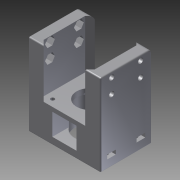
# Autodesk Inventor part: V5 Z Top
Saved by Autodesk Inventor 2012 (Build 160160000, 160)
## iProperties
Created: 2013-01-29
Part Number: V5 Z Top
Material: Default
Document SubType Name: Modeling
Designer: mce
Density: 1 g/cm^3
Author: mce
Autodesk Inventor part; units mm, degrees
ref_plane "YZ Plane" through (0, 0, 0) normal (1, 0, 0) x (0, 1, 0)
ref_plane "XZ Plane" through (0, 0, 0) normal (0, 1, 0) x (-1, 0, 0)
ref_plane "XY Plane" through (0, 0, 0) normal (0, 0, 1) x (1, 0, 0)
sketch "Sketch1" plane through (0, 0, 0) normal (0, 0, 1) x (1, 0, 0)
  line L0 (0, 0) -> (60, 0)
  line L1 (60, 0) -> (60, 42.4)
  line L2 (60, 42.4) -> (0, 42.4)
  line L3 (0, 42.4) -> (0, 0)
  line L4 (30, 50.4124) -> (30, -35.7574) construction
  line L5 (-22.9402, 21.2) -> (92.246, 21.2) construction
  circle A0 centre (30, 21.2) radius 11.1
  circle A1 centre (14.5, 36.7) radius 1.55
  circle A2 centre (45.5, 36.7) radius 1.55
  circle A3 centre (45.5, 5.7) radius 1.55
  circle A4 centre (14.5, 5.7) radius 1.55
  dimension "d0" = 60
  dimension "d1" = 42.4
  dimension "d2" = 22.2
  dimension "d3" = 3.1
  dimension "d4" = 31
  dimension "d5" = 31
  constraints: 12 end point, 5 centre point, 4 symmetric about line, 3 equal radius, 3 horizontal, 3 vertical, 2 point on line, 2 other
  measures "d0" distance of L0.start L0.end
  measures "d1" distance of L2.end L0.start
  measures "d2" diameter of A0
  measures "d3" diameter of A1
  measures "d4" distance of A4.centre A1.centre
  measures "d5" distance of A1.centre A2.centre
extrude "Extrusion1" add sketch "Sketch1" along normal blind 68
sketch "Sketch2" plane through (0, 0, 68) normal (0, 0, 1) x (1, 0, 0)
  circle A0 centre (30, 21.2) radius 11.1 projected
  circle A1 centre (14.5, 5.7) radius 1.55 projected
  circle A2 centre (45.5, 5.7) radius 1.55 projected
  circle A3 centre (45.5, 36.7) radius 1.55 projected
  circle A4 centre (14.5, 36.7) radius 1.55 projected
  line L0 (60, 0) -> (0, 0) projected
  line L1 (0, 42.4) -> (60, 42.4) projected
  line L2 (12.8, 42.4) -> (47.2, 42.4)
  line L3 (51.2, 38.4) -> (51.2, 4)
  line L4 (47.2, 0) -> (12.8, 0)
  line L5 (8.8, 4) -> (8.8, 38.4)
  line L6 (8.8, 38.4) -> (12.8, 42.4)
  line L7 (47.2, 42.4) -> (51.2, 38.4)
  line L8 (12.8, 0) -> (8.8, 4)
  line L9 (51.2, 4) -> (47.2, 0)
  point P0 (8.8, 42.4)
  point P1 (51.2, 0)
  point P2 (51.2, 42.4)
  point P3 (8.8, 0)
  dimension "d8" = 42.4
  dimension "d9" = 21.2
  dimension "d10" = 4
  dimension "d11" = 4
  dimension "d12" = 4
  dimension "d13" = 4
  dimension "d14" = 4
  dimension "d15" = 4
  dimension "d16" = 4
  dimension "d17" = 4
  constraints: 16 end point, 10 point on line
  measures "d8" distance between parallel lines of L5 L3
  measures "d9" distance from line of L5 A0.centre
  measures "d10" distance of L5.end point (8.8, 42.4)
  measures "d11" distance of L2.start point (8.8, 42.4)
  measures "d12" distance of L2.end point (51.2, 42.4)
  measures "d13" distance of L3.start point (51.2, 42.4)
  measures "d14" distance of L4.end point (8.8, 0)
  measures "d15" distance of L5.start point (8.8, 0)
  measures "d16" distance of L3.end point (51.2, 0)
  measures "d17" distance of L4.start point (51.2, 0)
extrude "Extrusion2" cut sketch "Sketch2" against normal blind 40.5
sketch "Sketch3" plane through (0, 0, 0) normal (-1, 0, 0) x (0, 0, 1)
  line L0 (68, 0) -> (68, 42.4) projected
  line L1 (0, 42.4) -> (68, 42.4) projected
  line L2 (0, 0) -> (68, 0) projected
  circle A0 centre (52, 33.2) radius 2.1
  circle A1 centre (64, 33.2) radius 2.1
  circle A2 centre (52, 9.2) radius 2.1
  circle A3 centre (64, 9.2) radius 2.1
  dimension "d20" = 4.2
  dimension "d21" = 12
  dimension "d22" = 12
  dimension "d23" = 4
  dimension "d24" = 9.2
  dimension "d25" = 9.2
  dimension "d26" = 4
  dimension "d27" = 9.2
  dimension "d28" = 9.2
  constraints: 4 centre point, 3 equal radius
  measures "d20" diameter of A0
  measures "d21" distance of A1.centre A0.centre
  measures "d22" distance of A2.centre A3.centre
  measures "d23" distance from line of L0 A1.centre
  measures "d24" distance from line of L1 A1.centre
  measures "d25" distance from line of L1 A0.centre
  measures "d26" distance from line of L0 A3.centre
  measures "d27" distance from line of L2 A3.centre
  measures "d28" distance from line of L2 A2.centre
extrude "Extrusion3" cut sketch "Sketch3" against normal through all
sketch "Sketch4" plane through (8.8, 4, 68) normal (1, 0, 0) x (0, 0, -1)
  circle A0 centre (4, 5.2) radius 2.1 projected
  circle A1 centre (16, 5.2) radius 2.1 projected
  circle A2 centre (4, 29.2) radius 2.1 projected
  circle A3 centre (16, 29.2) radius 2.1 projected
  line L0 (16, 25.1008) -> (12.45, 27.1504)
  line L1 (12.45, 27.1504) -> (12.45, 31.2496)
  line L2 (12.45, 31.2496) -> (16, 33.2992)
  line L3 (16, 33.2992) -> (19.55, 31.2496)
  line L4 (19.55, 31.2496) -> (19.55, 27.1504)
  line L5 (19.55, 27.1504) -> (16, 25.1008)
  line L6 (4, 25.1008) -> (0.45, 27.1504)
  line L7 (0.45, 27.1504) -> (0.45, 31.2496)
  line L8 (0.45, 31.2496) -> (4, 33.2992)
  line L9 (4, 33.2992) -> (7.55, 31.2496)
  line L10 (7.55, 31.2496) -> (7.55, 27.1504)
  line L11 (7.55, 27.1504) -> (4, 25.1008)
  line L12 (7.55, 3.1504) -> (4, 1.1008)
  line L13 (4, 1.1008) -> (0.45, 3.1504)
  line L14 (0.45, 3.1504) -> (0.45, 7.2496)
  line L15 (0.45, 7.2496) -> (4, 9.2992)
  line L16 (4, 9.2992) -> (7.55, 7.2496)
  line L17 (7.55, 7.2496) -> (7.55, 3.1504)
  line L18 (19.55, 3.1504) -> (16, 1.1008)
  line L19 (16, 1.1008) -> (12.45, 3.1504)
  line L20 (12.45, 3.1504) -> (12.45, 7.2496)
  line L21 (12.45, 7.2496) -> (16, 9.2992)
  line L22 (16, 9.2992) -> (19.55, 7.2496)
  line L23 (19.55, 7.2496) -> (19.55, 3.1504)
  point P0 (68, -4)
  point P1 (2.225, 26.1256)
  point P2 (12.45, 29.2)
  dimension "d31" = 7.1
  constraints: 48 end point, 4 coincident, 4 vertical, 3 equal length, 2 midpoint, 52 other
  measures "d31" distance between parallel lines of L16 L13
extrude "Extrusion4" cut sketch "Sketch4" against normal blind 5 and the other way blind 47.4
sketch "Sketch5" plane through (0, 1, 0) normal (-1, 0, 0) x (0, 0, 1)
  line L0 (0, 41.4) -> (0, -1) projected
  line L1 (7, 36) -> (10.5, 36)
  line L2 (10.5, 36) -> (10.5, 28.8)
  line L3 (10.5, 28.8) -> (7, 28.8)
  line L4 (7, 28.8) -> (7, 36)
  line L5 (7, 11.6) -> (10.5, 11.6)
  line L6 (10.5, 11.6) -> (10.5, 4.4)
  line L7 (10.5, 4.4) -> (7, 4.4)
  line L8 (7, 4.4) -> (7, 11.6)
  line L9 (0, 41.4) -> (68, 41.4) projected
  line L10 (68, 41.4) -> (27.5, 41.4) projected
  dimension "d37" = 7.2
  dimension "d38" = 3.5
  dimension "d39" = 24.4
  dimension "d41" = 7
  dimension "d105" = 5.4
  constraints: 16 end point, 4 vertical, 2 equal length, 2 horizontal, 1 collinear
  measures "d37" distance of L3.end L1.start
  measures "d38" distance of L1.start L1.end
  measures "d39" distance between parallel lines of L7 L3
  measures "d41" distance between parallel lines of L4 L0
  measures "d105" distance between parallel lines of L10 L1
extrude "Extrusion5" cut sketch "Sketch5" against normal blind 12
sketch "Sketch6" plane through (60, 1, 0) normal (1, 0, 0) x (0, 0, -1)
  line L0 (0, -1) -> (0, 41.4) projected
  line L1 (-10.5, 36) -> (-7, 36)
  line L2 (-7, 36) -> (-7, 28.8)
  line L3 (-7, 28.8) -> (-10.5, 28.8)
  line L4 (-10.5, 28.8) -> (-10.5, 36)
  line L5 (-10.5, 11.6) -> (-7, 11.6)
  line L6 (-7, 11.6) -> (-7, 4.4)
  line L7 (-7, 4.4) -> (-10.5, 4.4)
  line L8 (-10.5, 4.4) -> (-10.5, 11.6)
  line L9 (0, 41.4) -> (-68, 41.4) projected
  dimension "d44" = 3.5
  dimension "d45" = 7.2
  dimension "d46" = 7
  dimension "d47" = 24.4
  dimension "d67" = 5.4
  constraints: 16 end point, 4 horizontal, 4 vertical, 2 equal length, 1 collinear
  measures "d44" distance of L1.start L1.end
  measures "d45" distance of L1.end L2.end
  measures "d46" distance between parallel lines of L0 L2
  measures "d47" distance between parallel lines of L3 L7
  measures "d67" distance between parallel lines of L9 L1
extrude "Extrusion6" cut sketch "Sketch6" against normal blind 12
sketch "Sketch7" plane through (0, 0, 0) normal (0, 0, -1) x (-1, 0, 0)
  line L0 (-60, 0) -> (-60, 42.4) projected
  line L1 (0, 0) -> (-60, 0) projected
  line L2 (0, 42.4) -> (0, 0) projected
  line L3 (-60, 42.4) -> (0, 42.4) projected
  circle A0 centre (-55, 33.4) radius 2.05
  circle A1 centre (-5, 33.4) radius 2.05
  circle A2 centre (-5, 9) radius 2.05
  circle A3 centre (-55, 9) radius 2.05
  point P0 (-59, 42.4)
  point P1 (-60, 41.4)
  point P2 (-60, 1)
  point P3 (-59, 0)
  point P4 (-1, 0)
  point P5 (0, 1)
  point P6 (0, 41.4)
  point P7 (-1, 42.4)
  dimension "d51" = 5
  dimension "d52" = 5
  dimension "d53" = 5
  dimension "d54" = 5
  dimension "d55" = 9
  dimension "d56" = 9
  dimension "d57" = 9
  dimension "d58" = 9
  dimension "d59" = 4.1
  constraints: 4 centre point, 3 equal radius
  measures "d51" distance from line of L0 A0.centre
  measures "d52" distance from line of L0 A3.centre
  measures "d53" distance from line of L2 A2.centre
  measures "d54" distance from line of L2 A1.centre
  measures "d55" distance from line of L3 A0.centre
  measures "d56" distance from line of L1 A3.centre
  measures "d57" distance from line of L1 A2.centre
  measures "d58" distance from line of L3 A1.centre
  measures "d59" diameter of A0
extrude "Extrusion7" cut sketch "Sketch7" against normal blind 15 contours A0 | A1 | A2 | A3
sketch "Sketch8" plane through (0, 0, 0) normal (0, 0, -1) x (-1, 0, 0)
  circle A0 centre (-14.5, 5.7) radius 1.55 projected
  circle A1 centre (-45.5, 5.7) radius 1.55 projected
  circle A2 centre (-45.5, 36.7) radius 1.55 projected
  circle A3 centre (-14.5, 36.7) radius 1.55 projected
  circle A4 centre (-45.5, 36.7) radius 3
  circle A5 centre (-14.5, 36.7) radius 3
  circle A6 centre (-14.5, 5.7) radius 3
  circle A7 centre (-45.5, 5.7) radius 3
  point P0 (0, 0)
  dimension "d62" = 6
  constraints: 4 centre point, 4 coincident, 3 equal radius
  measures "d62" diameter of A4
extrude "Extrusion8" cut sketch "Sketch8" against normal blind 18
chamfer "Chamfer1" distance 3 angle 45 4 edges at (12, 12.6, 8.75) (12, 29.8, 8.75) (48, 29.8, 8.75) (48, 12.6, 8.75)
fillet "Fillet5" radius 3 2 edges at (53.6, 42.4, 68) (6.4, 42.4, 68)
fillet "Fillet3" radius 1 4 edges at (30, 42.4, 0) (60, 21.2, 0) (30, 0, 0) (0, 21.2, 0)
fillet "Fillet4" radius 1 10 edges at (60, 42.4, 33) (59.7071, 42.1071, 0.2929) (0.2929, 42.1071, 0.2929) (0, 42.4, 33) (59.7071, 0.2929, 0.2929) (60, 0, 34.5) (0.2929, 0.2929, 0.2929) (0, 0, 34.5) (53.6, 0, 68) (6.4, 0, 68)
sketch "Sketch9" plane through (12.8, 42.4, 27.5) normal (0, 1, 0) x (1, 0, 0)
  line L0 (7.2, 21.5) -> (27.2, 21.5)
  line L1 (27.2, 21.5) -> (27.2, 3.5)
  line L2 (27.2, 3.5) -> (7.2, 3.5)
  line L3 (7.2, 3.5) -> (7.2, 21.5)
  line L4 (-12.8, 26.5) -> (-12.8, -37.5) projected
  line L5 (46.2, 27.5) -> (-11.8, 27.5) projected
  point P0 (-12.8, 27.5)
  dimension "d74" = 18
  dimension "d75" = 20
  dimension "d76" = 20
  dimension "d77" = 6
  constraints: 8 end point, 1 horizontal, 1 vertical
  measures "d74" distance of L2.end L0.start
  measures "d75" distance of L1.end L2.end
  measures "d76" distance between parallel lines of L4 L3
  measures "d77" distance between parallel lines of L5 L0
extrude "Extrusion9" cut sketch "Sketch9" against normal through all
fillet "Fillet6" radius 2 2 edges at (30, 10.1, 6) (30, 32.3, 6)
sketch "Sketch10" plane through (0, 0, 0) normal (0, 0, -1) x (-1, 0, 0)
  circle A0 centre (-30, 21.2) radius 11.1 projected
  circle A1 centre (-30, 21.2) radius 12.5
  point P0 (0, 0)
  dimension "d85" = 25
  constraints: 1 centre point, 1 coincident
  measures "d85" diameter of A1
extrude "Extrusion10" cut sketch "Sketch10" against normal blind 23
fillet "Fillet8" radius 1 1 edges at (42.5, 21.2, 0)
sketch "Sketch11" plane through (0, 5.4, 10.5) normal (0, 0, -1) x (-1, 0, 0)
  circle A0 centre (-5, 3.6) radius 2.05 projected
  circle A1 centre (-5, 3.6) radius 2.05
  circle A2 centre (-5, 28) radius 2.05
  circle A3 centre (-55, 28) radius 2.05
  circle A4 centre (-55, 3.6) radius 2.05
  circle A5 centre (-55, 28) radius 2.05 projected
  circle A6 centre (-55, 3.6) radius 2.05 projected
  circle A7 centre (-5, 28) radius 2.05 projected
  point P0 (0, -5.4)
  constraints: 8 concentric, 4 centre point
extrude "Extrusion11" add sketch "Sketch11" against normal blind 0.2
sketch "Sketch12" plane through (45.5, 36.7, 18) normal (0, 0, -1) x (-1, 0, 0)
  circle A0 centre (0, 0) radius 1.55 projected
  circle A1 centre (0, 0) radius 1.55
  circle A2 centre (31, 0) radius 1.55
  circle A3 centre (31, -31) radius 1.55
  circle A4 centre (0, -31) radius 1.55
  circle A5 centre (31, 0) radius 1.55 projected
  circle A6 centre (31, -31) radius 1.55 projected
  circle A7 centre (0, -31) radius 1.55 projected
  point P0 (45.5, -36.7)
  constraints: 8 concentric, 4 centre point
extrude "Extrusion12" add sketch "Sketch12" against normal blind 0.2
sketch "Sketch13" plane through (40, 39.4, 24) normal (0, 0, -1) x (-1, 0, 0)
  arc A0 (0, -10.7) -> (20, -25.7) centre (10, -18.2) ccw projected
  line L0 (20, 0) -> (20, -36.4) projected
  line L1 (0, 0) -> (0, -36.4) projected
  line L2 (0, -10.7) -> (20, -10.7)
  line L3 (20, -10.7) -> (20, 85.3667)
  line L4 (20, 85.3667) -> (0, 7.3711)
  line L5 (0, 7.3711) -> (0, -10.7)
  line L6 (0, -25.7) -> (20, -25.7)
  line L7 (20, -25.7) -> (20, -66.8781)
  line L8 (20, -66.8781) -> (0, -69.4039)
  line L9 (0, -69.4039) -> (0, -25.7)
  line L10 (20, -25.7) -> (20, -36.4) projected
  line L11 (0, -10.7) -> (0, -36.4) projected
  point P0 (40, -39.4)
  constraints: 16 end point, 4 point on line, 2 coincident
equation "\"d5\" = d4"
equation "\"d9\" = 0.5 * d8"
equation "\"d11\" = d10"
equation "\"d12\" = d10"
equation "\"d13\" = d12"
equation "\"d14\" = d10"
equation "\"d15\" = d14"
equation "\"d16\" = d10"
equation "\"d17\" = d16"
body "Solid1"
